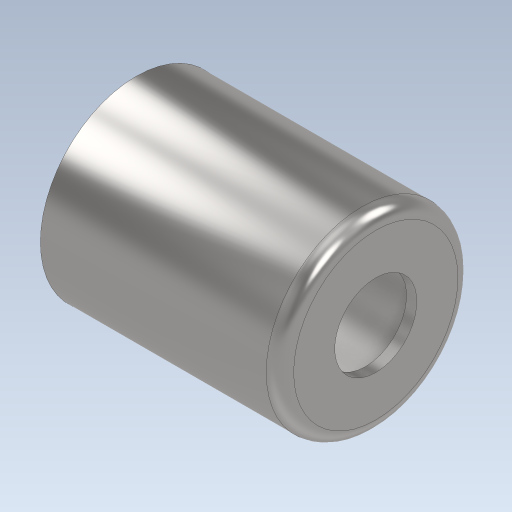
# Autodesk Inventor part: Pump-Motor-CW-Rotation:Cap 102
Saved by Autodesk Inventor 2024.2 (Build 282272000, 272)
## iProperties
Created: 2025-06-16
Material: Steel, Mild
Document SubType Name: Modeling
Density: 7.85 g/cm^3
Appearance: Semi-Polished
Designer: cw
Author: cw
Autodesk Inventor part; units mm, degrees
ref_plane "YZ Plane" through (0, 0, 0) normal (1, 0, 0) x (0, 1, 0)
ref_plane "XZ Plane" through (0, 0, 0) normal (0, 1, 0) x (-1, 0, 0)
ref_plane "XY Plane" through (0, 0, 0) normal (0, 0, 1) x (1, 0, 0)
sketch "Sketch1" plane through (0, 0, 0) normal (1, 0, 0) x (0, 1, 0)
  circle A0 centre (0, 0) radius 14
  dimension "d0" = 28
  constraints: 1 centre point, 1 coincident
  measures "d0" diameter of A0
extrude "Extrusion1" add sketch "Sketch1" against normal blind 35
shell "Shell1" thickness 1.5 removed faces 1 at (-35, 2.651, 3.8406)
sketch "Sketch2" plane through (0, 0, 0) normal (1, 0, 0) x (0, 0, -1)
  point P0 (0, 0)
hole "Hole1" at (0, 0, 0) direction (-1, 0, 0) diameter 12 end through all
fillet "Fillet1" radius 2 2 edges at (0, -14, 0) (-1.5, -12.5, 0)
body "Solid1"
